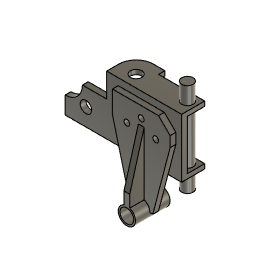
Tarea 10_jaalobuela (Autodesk Fusion 360 design; units mm, degrees)
Autodesk Fusion 360 part; units mm, degrees
sketch "Sketch9" plane through (0, 0, 0) normal (0, 1, 0) x (1, 0, 0)
  line L0 (200, -100) -> (200, -60)
  circle A0 through (234, -60, 0) (183, -60, -29.4449) (183, -60, 29.4449)
  circle A1 through (220, -100, 0) (190, -100, -17.3205) (190, -100, 17.3205)
  line L1 (200, -60) -> (166, -60)
  line L2 (200, -100) -> (180, -100)
  dimension "d51" = 68
  dimension "d52" = 40
  constraint coincident L0.end L1.start
  constraint coincident L0.start L2.start
cylinder "CylinderPrimitive4" add diameter 30 height 60 placed x (1, 0, 0) y (0, 0, -1) z (0, 1, 0) at (58.2159, 0, 70.3999) makes body 1
shell "Shell2" thickness 3 removed faces 2 at (62.3471, 0, 71.9221) at (62.3471, 60, 71.9221) on bodies 1
move_body "Move12" bodies 1 to x (1, 0, 0) y (0, 1, 0) z (0, 0, 1) at (171.7841, 0, -26.3999)
move_body "Move13" bodies 1 to x (1, 0, 0) y (0, 1, 0) z (0, 0, 1) at (0, -25, 0)
box "BoxPrimitive7" add length 108 width 25 height 10 placed x (0, 0, -1) y (0, 1, 0) z (1, 0, 0) at (0, 150, 175) separate body makes body 2
chamfer "Chamfer6" distance 88 distance2 25 1 edges at (5, 150, 175) measured on face at (3.3333, 150, 103) on bodies 2
move_body "Move14" bodies 2 to x (1, 0, 0) y (0, 1, 0) z (0, 0, 1) at (225, -175, -23)
move_body "Move15" bodies 2 to x (1, 0, 0) y (0, 1, 0) z (0, 0, 1) at (0, 0, 15)
combine "Combine2" operation add target body 2 tool bodies 1
box "BoxPrimitive8" add length 153 width 100 height 10 placed x (0, 0, -1) y (-1, 0, 0) z (0, 1, 0) at (60, 0, 110) separate body makes body 3
chamfer "Chamfer7" distance 115 distance2 30 1 edges at (-40, 5, -43) measured on face at (-40, 3.3333, 59) on bodies 3
chamfer "Chamfer8" distance 20 distance2 20 1 edges at (60, 5, 110) measured on face at (60, 3.3333, 59) on bodies 3
chamfer "Chamfer9" distance 30 distance2 115 1 edges at (60, 5, -43) measured on face at (36.6667, 3.3333, -43) on bodies 3
move_body "Move16" bodies 3 to x (1, 0, 0) y (0, 1, 0) z (0, 0, 1) at (108.3, 0, 0)
cylinder "CylinderPrimitive5" add diameter 30 height 47.845 placed x (1, 0, 0) y (0, 0, -1) z (0, 1, 0) at (20, 0, 5) separate body makes body 4
move_body "Move17" bodies 4 to x (1, 0, 0) y (0, 1, 0) z (0, 0, 1) at (98.3, 0, -48)
combine "Combine3" operation cut target body 3 tool bodies 4
move_body "Move18" bodies 3 to x (1, 0, 0) y (0, 1, 0) z (0, 0, 1) at (111.7, -25, 87)
move_body "Move19" bodies 3 to x (1, 0, 0) y (0, 1, 0) z (0, 0, 1) at (0, 25, 0)
sketch "Sketch15" plane through (0, 0, 0) normal (0, 1, 0) x (1, 0, 0)
  line L0 (92, -95) -> (222, -95)
  line L1 (222, -95) -> (222, 7)
  line L2 (222, 7) -> (20, 7)
  line L3 (20, 7) -> (20, -53)
  line L4 (20, -53) -> (50, -53)
  line L5 (50, -53) -> (92, -53)
  line L6 (92, -53) -> (92, -95)
  dimension "d133" = 102
  dimension "d134" = 202
  dimension "d135" = 60
  dimension "d136" = 30
  dimension "d137" = 42
  constraint perpendicular L0 L1
  constraint perpendicular L1 L2
  constraint perpendicular L0 L3
  constraint perpendicular L3 L4
  constraint perpendicular L0 L6
  measures "d133" distance of L0.end L1.end
  measures "d134" distance of L1.end L2.end
  measures "d135" distance of L2.end L3.end
  measures "d136" distance of L3.end L4.end
  measures "d137" distance of L4.end L5.end
extrude "Extrude2" add sketch "Sketch15" along normal blind 10 separate body makes body 5
move_body "Move20" bodies 5 to x (1, 0, 0) y (0, 1, 0) z (0, 0, 1) at (0, -110, 0)
cylinder "CylinderPrimitive6" add diameter 60 height 10 placed x (1, 0, 0) y (0, 0, -1) z (0, 1, 0) at (-60, 0, 110) separate body makes body 6
move_body "Move21" bodies 6 to x (1, 0, 0) y (0, 1, 0) z (0, 0, 1) at (80, -110, -57)
combine "Combine4" operation cut target body 5 tool bodies 6
hole "Hole8" at (56, -110, 23) direction (0, 1, 0) diameter 20 depth 60 tip angle 118 bodies 5
move_body "Move22" bodies 5 to x (1, 0, 0) y (0, 1, 0) z (0, 0, 1) at (63, 120, 102)
move_body "Move23" bodies 5 to x (1, 0, 0) y (0, 1, 0) z (0, 0, 1) at (0, 0, 12)
sketch "Sketch17" plane through (0, 0, 0) normal (0, 0, 1) x (1, 0, 0)
  line L0 (240, 150) -> (370, 150)
  line L1 (370, 150) -> (370, 99)
  line L2 (370, 99) -> (240, 99)
  line L3 (240, 99) -> (240, 150)
  dimension "d153" = 51
  dimension "d154" = 130
  constraint horizontal L0
  constraint vertical L1
  constraint horizontal L2
  constraint vertical L3
  measures "d153" distance of L0.start L2.end
  measures "d154" distance of L0.start L0.end
extrude "Extrude3" add sketch "Sketch17" along normal blind 8 separate body makes body 7
box "BoxPrimitive9" add length 11 width 80 height 10 placed x (0, -1, 0) y (1, 0, 0) z (0, 0, 1) at (306.4018, 216.5557, 0) separate body makes body 8
move_body "Move24" bodies 8 to x (1, 0, 0) y (0, 1, 0) z (0, 0, 1) at (-16.4018, -66.5557, 0)
combine "Combine5" operation cut target body 7 tool bodies 8
fillet "Fillet3" radius 30 1 edges at (240, 150, 4) on bodies 7
hole "Hole9" at (270, 120, 8) direction (0, 0, -1) diameter 20 depth 60 tip angle 118 bodies 7
move_body "Move25" bodies 7 to x (1, 0, 0) y (0, 1, 0) z (0, 0, 1) at (-85, -89, 201)
hole "Hole10" at (270, 35, 209) direction (0, 0, -1) diameter 20 depth 60 tip angle 118 bodies 7
copy_body "CopyPasteBodies2" bodies 7 makes body 9
move_body "Move27" bodies 9 to x (1, 0, 0) y (0, 1, 0) z (0, 0, 1) at (0, 0, -94)
cylinder "CylinderPrimitive7" add diameter 20 height 162 placed x (1, 0, 0) y (0, 1, 0) z (0, 0, 1) at (20, 20, 0) separate body makes body 10
move_body "Move28" bodies 10 to x (1, 0, 0) y (0, 1, 0) z (0, 0, 1) at (250, 15, 47)
move_body "Move29" bodies 10 to x (1, 0, 0) y (0, 1, 0) z (0, 0, 1) at (0, 0, 30)
copy_body "CopyPasteBodies3" bodies 2 9 5 10 7 3 makes body 11 makes body 12 makes body 13 makes body 14 makes body 15 makes body 16
move_body "Move30" bodies 11 12 13 14 15 16 to x (1, 0, 0) y (0, 1, 0) z (0, 0, 1) at (250, 0, 0)
move_body "Move31" bodies 16 11 to x (1, 0, 0) y (0, 1, 0) z (0, 0, 1) at (-5, 0, 0)
combine "Combine6" operation add target body 12 tool bodies 16 11 14 15 13
hole "Hole11" at (500, 0, 159) direction (0, 1, 0) diameter 10 depth 60 tip angle 118 bodies 12
hole "Hole12" at (475, 0, 178) direction (0, 1, 0) diameter 10 depth 60 tip angle 118 bodies 12
hole "Hole13" at (450, 0, 159) direction (0, 1, 0) diameter 10 depth 60 tip angle 118 bodies 12
extrude "Extrude4" add 1 faces at (476.6667, -16.6667, 59) along direction (0, 0, -1) blind 2 on bodies 12 bodies 12
extrude "Extrude5" add 1 faces at (471.6667, -8.3333, 59) along direction (0, 0, -1) blind 2 on bodies 12 bodies 12
hidden bodies 2 3 5 7 9 10
